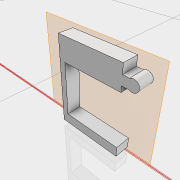
# Autodesk Inventor part: ЛЦМК.00002.00.00.00.00.22 Крышка короба
Saved by Autodesk Inventor 2021.2 (Build 252289000, 289)
## iProperties
Created: 2025-11-20
Part Number: ЛЦМК.00002.00.00.00.00.22 Крышка короба
Material: Типовые
Document SubType Name: Modeling
Designer: Захаров
Density: 1 g/cm^3
Appearance: По умолчанию
Author: Захаров
Autodesk Inventor part; units mm, degrees
ref_plane "YZ Plane" through (0, 0, 0) normal (1, 0, 0) x (0, 1, 0)
ref_plane "XZ Plane" through (0, 0, 0) normal (0, 1, 0) x (-1, 0, 0)
ref_plane "XY Plane" through (0, 0, 0) normal (0, 0, 1) x (1, 0, 0)
ref_plane "РабПлоскость1" through (0, 0, 0) normal (0, 0, 1) x (1, 0, 0)
sketch "Эскиз1" plane through (0, 0, 0) normal (0, 0, 1) x (1, 0, 0)
  arc A0 (-52.0649, -23.6861) -> (-52.0649, -20.6861) centre (-51.0649, -22.1861) ccw
  line L0 (-52.0649, -23.6861) -> (-54.0649, -23.6861)
  line L1 (-54.0649, -20.6861) -> (-52.0649, -20.6861)
  line L2 (-54.0649, -17.6861) -> (-54.0649, -20.6861)
  line L3 (-73.5649, -42.0009) -> (-52.0649, -42.0009)
  line L4 (-52.0649, -24.0009) -> (-73.5649, -24.0009)
  line L5 (-73.5649, -24.0009) -> (-73.5649, -42.0009)
  line L6 (-75.5649, -28.2509) -> (-75.5649, -37.7509)
  line L7 (-54.0649, -17.6861) -> (-75.5649, -17.6861)
  line L8 (-75.5649, -17.6861) -> (-75.5649, -28.2509)
  line L9 (-75.5649, -37.7509) -> (-75.5649, -45.4011)
  line L10 (-75.5649, -45.4011) -> (-75.4649, -45.4011)
  line L11 (-54.0649, -23.6861) -> (-54.0649, -24.0009)
  line L12 (-54.0649, -43.0726) -> (-54.0649, -42.0009)
  line L13 (-54.0649, -43.0726) -> (-75.5649, -43.0726)
  line L14 (-54.1649, -24.0009) -> (-54.1649, -23.5861)
  line L15 (-54.1649, -23.5861) -> (-52.0341, -23.5861)
  arc A1 (-52.0341, -23.5861) -> (-52.0341, -20.7861) centre (-51.0649, -22.1861) ccw
  line L16 (-52.0341, -20.7861) -> (-54.1649, -20.7861)
  line L17 (-54.1649, -20.7861) -> (-54.1649, -17.7861)
  line L18 (-54.1649, -17.7861) -> (-75.4649, -17.7861)
  line L19 (-75.4649, -17.7861) -> (-75.4649, -28.2509)
  line L20 (-75.4649, -28.2509) -> (-75.4649, -37.7509)
  line L21 (-75.4649, -37.7509) -> (-75.4649, -43.0726)
  point P0 (0, 0)
extrude "Выдавливание1" add sketch "Эскиз1" against normal blind 5
